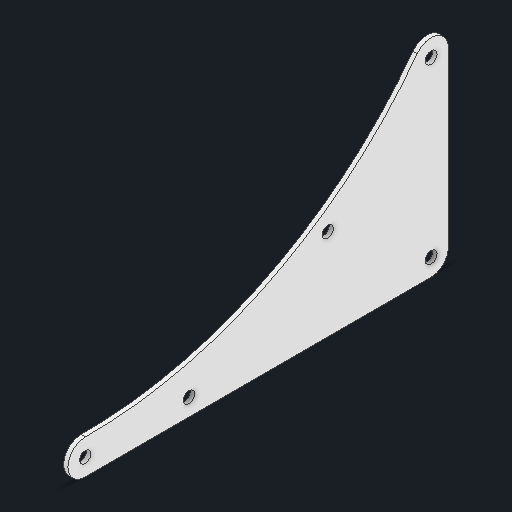
# Autodesk Inventor part: Scoop Gusset
Saved by Autodesk Inventor 2025.1 (Build 291241000, 241)
## iProperties
Created: 2024-10-25
Part Number: Scoop Gusset
Material: Acetal Resin, White
Document SubType Name: Modeling
Designer: avere
Density: 1.425 g/cm^3
Appearance: Smooth - White
Author: avere
Autodesk Inventor part; units mm, degrees
ref_plane "YZ Plane" through (0, 0, 0) normal (1, 0, 0) x (0, 1, 0)
ref_plane "XZ Plane" through (0, 0, 0) normal (0, 1, 0) x (-1, 0, 0)
ref_plane "XY Plane" through (0, 0, 0) normal (0, 0, 1) x (1, 0, 0)
sketch "main" plane through (0, 0, 0) normal (0, 0, 1) x (1, 0, 0)
  circle A0 centre (-72.2021, -58.7899) radius 2.1844
  circle A1 centre (-8.7021, -58.7899) radius 2.1844
  circle A2 centre (-72.2021, 68.2101) radius 2.0955
  arc A3 (-65.8522, 68.1715) -> (-78.5521, 68.2101) centre (-72.2021, 68.2101) ccw
  arc A4 (-78.5521, -58.7899) -> (-72.2021, -65.1399) centre (-72.2021, -58.7899) ccw
  arc A5 (-8.7021, -65.1399) -> (-4.923, -53.6869) centre (-8.7021, -58.7899) ccw
  line L0 (-8.7021, -65.1399) -> (-72.2021, -65.1399)
  line L1 (-78.5521, -58.7899) -> (-78.5521, 68.2101)
  arc A6 (-65.8522, 68.1715) -> (-4.923, -53.6869) centre (84.6432, 67.2577) ccw
  circle A7 centre (-45.1241, -20.8434) radius 2.0955
  circle A8 centre (-72.2021, 30.1101) radius 2.0955
  point P0 (-46.4652, -14.2849)
  dimension "d0" = 4.191
  dimension "d1" = 12.7
  dimension "d3" = 4.191
  dimension "d4" = 4.191
  measures "d0" diameter of A2
  measures "d1" diameter of A5
  measures "d3" diameter of A7
  measures "d4" diameter of A8
sketch "Sketch1" plane through (0, 0, 0) normal (1, 0, 0) x (0, 1, 0)
  circle A0 centre (0, 0) radius 2.1844
  circle A1 centre (63.5, 0) radius 2.1844
  circle A2 centre (0, 127) radius 2.0955
  arc A3 (6.3499, 126.9614) -> (-6.35, 127) centre (0, 127) ccw
  arc A4 (-6.35, 0) -> (0, -6.35) centre (0, 0) ccw
  arc A5 (63.5, -6.35) -> (67.2791, 5.103) centre (63.5, 0) ccw
  line L0 (63.5, -6.35) -> (0, -6.35)
  line L1 (-6.35, 0) -> (-6.35, 127)
  arc A6 (6.3499, 126.9614) -> (67.2791, 5.103) centre (156.8453, 126.0476) ccw
  circle A7 centre (27.078, 37.9465) radius 2.0955
  circle A8 centre (0, 88.9) radius 2.0955
  constraints: 1 other
extrude "Extrusion1" add sketch "Sketch1" against normal blind 1.5875
body "Solid1"
